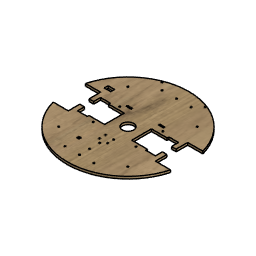
Bottom Plane (Autodesk Fusion 360 design; units mm, degrees)
Autodesk Fusion 360 part; units mm, degrees
sketch "Sketch1" plane through (0, 0, 0) normal (0, 0, 1) x (1, 0, 0)
  circle A0 centre (0, 0) radius 132
  line L0 (-29.5, 21.3) -> (-29.5, -21.3)
  line L1 (-94.5, -35) -> (-127.2753, -35)
  line L2 (-63.5, 21.3) -> (-29.5, 21.3)
  line L3 (-63.5, -21.3) -> (-29.5, -21.3)
  line L4 (-63.5, 25) -> (-84.5, 25)
  line L5 (-84.5, -25) -> (-63.5, -25)
  line L6 (-63.5, -25) -> (-63.5, -21.3)
  line L7 (-63.5, 21.3) -> (-63.5, 25)
  line L8 (-94.5, 35) -> (-127.2753, 35)
  circle A1 centre (-46.5, 29) radius 1.75
  circle A2 centre (-46.5, -29) radius 1.75
  line L9 (0, 2.5) -> (0, 20)
  circle A3 centre (8.75, -53) radius 1.75
  circle A4 centre (8.75, -40) radius 1.75
  circle A5 centre (-8.75, -40) radius 1.75
  circle A6 centre (-8.75, -53) radius 1.75
  line L10 (-124.5, -35) -> (-124.5, 35)
  line L11 (-84.5, -10) -> (-94.5, -10)
  line L12 (-84.5, 10) -> (-94.5, 10)
  line L13 (-84.5, 25) -> (-84.5, 10)
  line L14 (-84.5, -10) -> (-84.5, -25)
  line L15 (-94.5, -35) -> (-94.5, -10)
  line L16 (-94.5, 10) -> (-94.5, 35)
  line L17 (94.5, -35) -> (94.5, -10)
  line L18 (94.5, 10) -> (94.5, 35)
  circle A7 centre (46.5, 29) radius 1.75
  line L19 (63.5, 25) -> (84.5, 25)
  line L20 (94.5, 35) -> (127.2753, 35)
  line L21 (84.5, 25) -> (84.5, 10)
  line L22 (29.5, 21.3) -> (29.5, -21.3)
  line L23 (84.5, -10) -> (94.5, -10)
  line L24 (124.5, -35) -> (124.5, 35)
  line L25 (63.5, -25) -> (63.5, -21.3)
  line L26 (84.5, -10) -> (84.5, -25)
  line L27 (84.5, -25) -> (63.5, -25)
  line L28 (63.5, -21.3) -> (29.5, -21.3)
  line L29 (63.5, 21.3) -> (29.5, 21.3)
  line L30 (94.5, -35) -> (127.2753, -35)
  circle A8 centre (46.5, -29) radius 1.75
  line L31 (84.5, 10) -> (94.5, 10)
  line L32 (63.5, 21.3) -> (63.5, 25)
  line L33 (40.5, 36.3) -> (29.5, 36.3)
  line L34 (29.5, 36.3) -> (29.5, 39.3)
  line L35 (29.5, 39.3) -> (40.5, 39.3)
  line L36 (40.5, 39.3) -> (40.5, 36.3)
  line L37 (-40.5, 39.3) -> (-40.5, 36.3)
  line L38 (-40.5, 36.3) -> (-29.5, 36.3)
  line L39 (-29.5, 39.3) -> (-40.5, 39.3)
  line L40 (-29.5, 36.3) -> (-29.5, 39.3)
  line L41 (-84.5, 47) -> (-98.5, 47)
  line L42 (-98.5, 47) -> (-98.5, 55.4)
  line L43 (-98.5, 55.4) -> (-84.5, 55.4)
  line L44 (-84.5, 55.4) -> (-84.5, 47)
  circle A9 centre (0, -105.3) radius 1.75
  circle A10 centre (0, -83.3) radius 1.75
  circle A11 centre (0, -61.3) radius 1.75
  line L45 (-30, -76.3) -> (-35, -76.3)
  line L46 (-35, -76.3) -> (-35, -71.3)
  line L47 (-35, -71.3) -> (-30, -71.3)
  line L48 (-30, -71.3) -> (-30, -76.3)
  circle A12 centre (75, -75) radius 1.75
  circle A13 centre (75, 75) radius 1.75
  circle A14 centre (-75, 75) radius 1.75
  circle A15 centre (-75, -75) radius 1.75
  circle A16 centre (-31.5, -105.3) radius 1.75
  circle A17 centre (31.5, -105.3) radius 1.75
  circle A18 centre (-31.5, 105.3) radius 1.75
  circle A19 centre (31.5, 105.3) radius 1.75
  circle A20 centre (0, 105.3) radius 1.75
  circle A21 centre (-46.5, 120.5) radius 1.75
  circle A22 centre (46.5, 120.5) radius 1.75
  circle A23 centre (0, 0) radius 12.5
  point P0 (0, 80.767)
  point P1 (0, -132)
  point P2 (0, -83.3)
  point P3 (0, 74)
  dimension "d1" = 264
  dimension "d12" = 42.6
  dimension "d14" = 21.3
  dimension "d15" = 21
  dimension "d16" = 50
  dimension "d20" = 34
  dimension "d24" = 3.7
  dimension "d25" = 3.7
  dimension "d28" = 10
  dimension "d30" = 3.5
  dimension "d31" = 7.7
  dimension "d32" = 17
  dimension "d33" = 7.7
  dimension "d34" = 17
  dimension "d111" = 40
  dimension "d112" = 30
  dimension "d113" = 15
  dimension "d114" = 15
  dimension "d119" = 3.5
  dimension "d124" = 3.5
  dimension "d127" = 13
  dimension "d129" = 3.5
  dimension "d130" = 11
  dimension "d131" = 3
  dimension "d134" = 70
  dimension "d148" = 8.4
  dimension "d150" = 3.5
  dimension "d151" = 3.5
  dimension "d153" = 22
  dimension "d154" = 3.5
  dimension "d155" = 22
  dimension "d160" = 5
  dimension "d161" = 5
  dimension "d162" = 30
  dimension "d163" = 10
  dimension "d164" = 3.5
  dimension "d190" = 3.5
  dimension "d191" = 3.5
  dimension "d209" = 13
  dimension "d211" = 31.5
  dimension "d212" = 31.5
  dimension "d220" = 29.5
  dimension "d221" = 29.5
  dimension "d222" = 12
  dimension "d223" = 14
  dimension "d224" = 10
  dimension "d226" = 15
  dimension "d229" = 18.7
  dimension "d236" = 50
  dimension "d237" = 19.5
  dimension "d238" = 50
  dimension "d239" = 19.5
  dimension "d240" = 3.5
  dimension "d242" = 91.5
  dimension "d243" = 3.5
  dimension "d244" = 3.5
  dimension "d245" = 9.5
  dimension "d246" = 19.6
  dimension "d247" = 3.5
  dimension "d248" = 40
  dimension "d249" = 19.5
  dimension "d250" = 3.5
  dimension "d251" = 25
  dimension "d253" = 46.5
  dimension "d255" = 91.5
  dimension "d256" = 40
  dimension "d261" = 8.75
  dimension "d262" = 8.75
  dimension "d263" = 13
  dimension "d264" = 8.75
  dimension "d265" = 17.5
  dimension "d266" = 8.3
  dimension "d267" = 8.75
  dimension "d268" = 29
  dimension "d269" = 3.5
  dimension "d270" = 22
  constraint coincident A0.centre A23.centre
  constraint vertical L0
  constraint horizontal L1
  constraint perpendicular L0 L2
  constraint perpendicular L0 L3
  constraint horizontal L4
  constraint vertical L13
  constraint horizontal L5
  constraint vertical L6
  constraint collinear L6 L7
  constraint perpendicular L8 L13
  constraint equal A1 A2
  constraint perpendicular L8 L10
  constraint perpendicular L8 L15
  constraint coincident L11.start L13
  constraint perpendicular L11 L15
  constraint coincident L12.end L15
  constraint perpendicular L12 L15
  constraint collinear L13 L14
  constraint collinear L15 L16
  constraint symmetric L2.start L9 L29.start
  constraint symmetric L3.start L9 L25.end
  constraint symmetric L0.start L9 L22.start
  constraint symmetric L0.end L9 L22.end
  constraint symmetric L4.start L9 L19.start
  constraint symmetric L4.end L9 L19.end
  constraint symmetric L5.start L9 L26.end
  constraint symmetric L5.end L9 L25.start
  constraint symmetric A1 L9 A7
  constraint symmetric A2 L9 A8
  constraint symmetric L9 L10.start L24.start
  constraint symmetric L9 L10.end L24.end
  constraint symmetric L9 L1.start L17.start
  constraint symmetric L9 L8.start L18.end
  constraint symmetric L9 L11.start L23.start
  constraint symmetric L9 L11.end L17.end
  constraint symmetric L9 L12.start L21.end
  constraint symmetric L9 L12.end L18.start
  constraint equal A5 A6
  constraint horizontal L33
  constraint vertical L34
  constraint horizontal L35
  constraint vertical L36
  constraint symmetric L9 L33.start L37.end
  constraint symmetric L9 L33.end L38.end
  constraint symmetric L9 L34.end L39.start
  constraint symmetric L9 L35.end L37.start
  constraint horizontal L41
  constraint vertical L42
  constraint horizontal L43
  constraint vertical L44
  constraint collinear A9.centre P2 A11.centre
  constraint horizontal L45
  constraint vertical L46
  constraint horizontal L47
  constraint vertical L48
  constraint collinear L13 L44
  constraint coincident A0 P1
  constraint coincident P2 A10.centre
  constraint collinear L0 L40
  constraint concentric A0 A23
  constraint coincident A0 L8.end
  constraint coincident L8 L10.end
  constraint coincident A0 L1.end
  constraint coincident L1 L10.start
  constraint coincident A0 L30.end
  constraint coincident L24.start L30
  constraint coincident A0 L20.end
  constraint coincident L24.end L20
  measures "d1" diameter of A0
  measures "d12" distance of L2.start L3.start
  measures "d14" vertical distance of A0.centre L3.start
  measures "d15" distance of L4.start L4.end
  measures "d16" distance of L4.start L5.end
  measures "d20" distance of L0 L7
  measures "d24" distance of L2.start L4.start
  measures "d25" distance of L3.start L5.end
  measures "d28" distance of L4 L8
  measures "d30" diameter of A1
  measures "d31" distance of L2 A1.centre
  measures "d32" distance of L0 A1.centre
  measures "d33" distance of L3 A2.centre
  measures "d34" distance of L0 A2.centre
  measures "d111" distance of L10 L13
  measures "d112" distance of L10 L15
  measures "d113" distance of L5 L11
  measures "d114" distance of L4 L12
  measures "d119" diameter of A4
  measures "d124" diameter of A5
  measures "d127" distance of A3.centre A4.centre
  measures "d129" diameter of A3
  measures "d130" distance of L33.start L33.end
  measures "d131" distance of L33.start L35.end
  measures "d134" distance of L1 L8
  measures "d148" distance of L41.start L43.end
  measures "d150" diameter of A9
  measures "d151" diameter of A10
  measures "d153" distance of A9.centre P2
  measures "d154" diameter of A11
  measures "d155" distance of P2 A11.centre
  measures "d160" distance of L45.start L45.end
  measures "d161" distance of L45.start L47.end
  measures "d162" distance of A11.centre L48
  measures "d163" distance of A11.centre L47
  measures "d164" diameter of A12
  measures "d190" diameter of A16
  measures "d191" diameter of A17
  measures "d209" distance of A3.centre A4.centre
  measures "d211" distance of A9.centre A16.centre
  measures "d212" distance of A9.centre A17.centre
  measures "d220" distance of A0.centre L0
  measures "d221" distance of A0.centre L22
  measures "d222" distance of L8 L41
  measures "d223" distance of L42 L44
  measures "d224" distance of L14 L15
  measures "d226" distance of L2 L38
  measures "d229" distance of A4.centre L28
  measures "d236" distance of L27 A12.centre
  measures "d237" distance of L17 A12.centre
  measures "d238" distance of L5 A15.centre
  measures "d239" distance of L15 A15.centre
  measures "d240" diameter of A15
  measures "d242" distance of A1.centre A21.centre
  measures "d243" diameter of A21
  measures "d244" diameter of A22
  measures "d245" distance of L44 A14.centre
  measures "d246" distance of L43 A14.centre
  measures "d247" diameter of A14
  measures "d248" distance of L20 A13.centre
  measures "d249" distance of L18 A13.centre
  measures "d250" diameter of A13
  measures "d251" diameter of A23
  measures "d253" horizontal distance of A21.centre A0.centre
  measures "d255" distance of A7.centre A22.centre
  measures "d256" vertical distance of A5.centre A0.centre
  measures "d261" horizontal distance of A5.centre A0.centre
  measures "d262" horizontal distance of A4.centre A0.centre
  measures "d263" vertical distance of A6.centre A5.centre
  measures "d264" horizontal distance of A6.centre A0.centre
  measures "d265" distance of A3.centre A6.centre
  measures "d266" vertical distance of A3.centre A11.centre
  measures "d267" horizontal distance of A3.centre A11.centre
  measures "d268" distance of L45 A16.centre
  measures "d269" distance of L46 A16.centre
  measures "d270" vertical distance of P2 A17.centre
extrude "Extrude1" add sketch "Sketch1" along normal blind 5 contours A0 L0 L1 L2 L3 L4 L5 L6 L7 L8 L11 L12 L13 L14 L15 L16 L17 L18 L19 L20 L21 L22 L23 L25 L26 L27 L28 L29 L30 L31 L32
